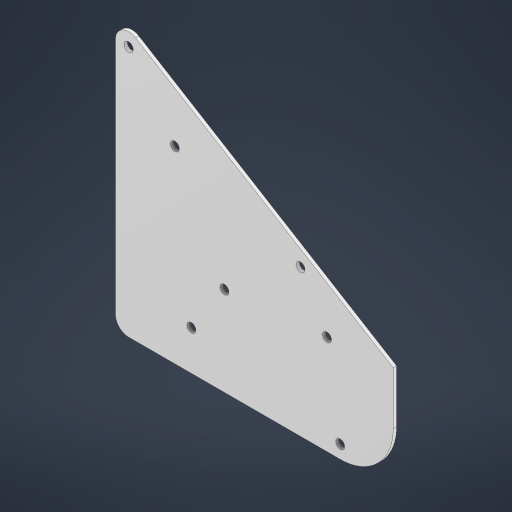
# Autodesk Inventor part: blocker
Saved by Autodesk Inventor 2024 (Build 280153000, 153)
## iProperties
Created: 2023-11-29
Part Number: blocker
Material: Acetal Resin, White
Document SubType Name: Sheet Metal
Designer: avere
Density: 1.425 g/cm^3
Appearance: Smooth - White
Flat Pattern Width: 11.0342 cm
Flat Pattern Length: 16.8058 cm
Flat Pattern Area: 185.439 cm^2
Sheet Metal Rule: Default_mm
Sheet Metal Width: 4.344 in
Sheet Metal Length: 6.616 in
Sheet Metal Area: 28.743 in^2
Author: avere
Autodesk Inventor part; units mm, degrees
ref_plane "YZ Plane" through (0, 0, 0) normal (1, 0, 0) x (0, 1, 0)
ref_plane "XZ Plane" through (0, 0, 0) normal (0, 1, 0) x (-1, 0, 0)
ref_plane "XY Plane" through (0, 0, 0) normal (0, 0, 1) x (1, 0, 0)
sketch "Block1" plane through (0, 0, 0) normal (0, 0, 1) x (1, 0, 0)
  circle A0 centre (36.7608, -51.6694) radius 2.0955
  circle A1 centre (30.4108, -10.3944) radius 2.0955
  circle A2 centre (17.7108, 12.3965) radius 2.0955
  circle A3 centre (-18.8017, -15.1569) radius 2.0955
  circle A4 centre (-34.6767, -38.9694) radius 2.0955
  line L0 (-64.8392, -58.0194) -> (36.7608, -58.0194)
  line L1 (62.1608, -7.2194) -> (-61.5382, 68.0552)
  circle A5 centre (-42.6142, 32.4681) radius 2.0955
  circle A6 centre (-64.8392, 62.6306) radius 2.1844
  arc A7 (-61.5382, 68.0552) -> (-71.1892, 62.6306) centre (-64.8392, 62.6306) ccw
  line L2 (-71.1892, -51.6694) -> (-71.1892, 62.6306)
  arc A8 (-71.1892, -51.6694) -> (-64.8392, -58.0194) centre (-64.8392, -51.6694) ccw
  line L3 (62.1608, -32.6194) -> (62.1608, -7.2194)
  arc A9 (36.7608, -58.0194) -> (62.1608, -32.6194) centre (36.7608, -32.6194) ccw
  point P0 (-13.0925, -13.6067)
  point P1 (62.1608, -58.0194)
  dimension "d0" = 12.7
  dimension "d1" = 12.7
  dimension "d2" = 50.8
  dimension "d3" = 25.4
  dimension "d4" = 4.191
  dimension "d5" = 4.191
  dimension "d6" = 4.191
  dimension "d7" = 4.191
  dimension "d8" = 4.191
  dimension "d9" = 4.191
  measures "d0" diameter of A8
  measures "d1" diameter of A7
  measures "d2" distance of point (62.161, -58.019) L3.end
  measures "d3" radius of A9
  measures "d4" diameter of A0
  measures "d5" diameter of A1
  measures "d6" diameter of A4
  measures "d7" diameter of A2
  measures "d8" diameter of A3
  measures "d9" diameter of A5
sketch "main" plane through (0, 0, 0) normal (0, 0, 1) x (1, 0, 0)
  circle A0 centre (36.7608, -51.6694) radius 2.0955
  circle A1 centre (30.4108, -10.3944) radius 2.0955
  circle A2 centre (17.7108, 12.3965) radius 2.0955
  circle A3 centre (-18.8017, -15.1569) radius 2.0955
  circle A4 centre (-34.6767, -38.9694) radius 2.0955
  line L0 (-64.8392, -58.0194) -> (36.7608, -58.0194)
  line L1 (62.1608, -7.2194) -> (-61.5382, 68.0552)
  circle A5 centre (-42.6142, 32.4681) radius 2.0955
  circle A6 centre (-64.8392, 62.6306) radius 2.1844
  arc A7 (-61.5382, 68.0552) -> (-71.1892, 62.6306) centre (-64.8392, 62.6306) ccw
  line L2 (-71.1892, -51.6694) -> (-71.1892, 62.6306)
  arc A8 (-71.1892, -51.6694) -> (-64.8392, -58.0194) centre (-64.8392, -51.6694) ccw
  line L3 (62.1608, -32.6194) -> (62.1608, -7.2194)
  arc A9 (36.7608, -58.0194) -> (62.1608, -32.6194) centre (36.7608, -32.6194) ccw
  point P0 (-13.0925, -13.6067)
sketch "Sketch1" plane through (0, 0, 0) normal (0, 0, 1) x (1, 0, 0)
  circle A0 centre (12.7, 0) radius 2.0955
  circle A1 centre (101.6, 0) radius 2.0955
  circle A2 centre (95.25, 41.275) radius 2.0955
  circle A3 centre (82.55, 64.0658) radius 2.0955
  circle A4 centre (46.0375, 36.5125) radius 2.0955
  circle A5 centre (30.1625, 12.7) radius 2.0955
  line L0 (0, -6.35) -> (101.6, -6.35)
  line L1 (127, 44.45) -> (3.301, 119.7246)
  circle A6 centre (22.225, 84.1375) radius 2.0955
  circle A7 centre (0, 114.3) radius 2.1844
  arc A8 (3.301, 119.7246) -> (-6.35, 114.3) centre (0, 114.3) ccw
  line L2 (-6.35, 0) -> (-6.35, 114.3)
  arc A9 (-6.35, 0) -> (0, -6.35) centre (0, 0) ccw
  line L3 (127, 19.05) -> (127, 44.45)
  arc A10 (101.6, -6.35) -> (127, 19.05) centre (101.6, 19.05) ccw
  dimension "d12" = 4.191
  constraints: 1 centre point, 1 other
  measures "d12" diameter of A0
extrude "Extrusion1" add sketch "Sketch1" along normal blind 1.5875 contours A0 | A9 L2 A8 L1 L3 A10 L0
equation "\"BendRadius\" = Thickness"
equation "\"BendReliefWidth\" = Thickness"
equation "\"BendReliefDepth\" = 0.5 * Thickness"
equation "\"CornerReliefSize\" = 4 * Thickness"
equation "\"MinimumRemnant\" = 2 * Thickness"
equation "\"TransitionRadius\" = BendRadius"
equation "\"JacobiRadiusSize\" = BendRadius"
equation "\"GapSize\" = Thickness"
equation "\"Thickness\" = 1.5875"
body "Solid1"
